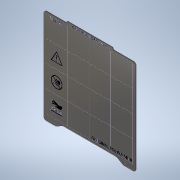
# Autodesk Inventor part: MINI-steel-sheet
Saved by Autodesk Inventor 2021 (Build 250183000, 183)
## iProperties
Created: 2019-07-15
Material: Všeobecné
Document SubType Name: Modeling
Density: 1 g/cm^3
Appearance: Ocel – leštěná
Project: ORIGINAL PRUSA MINI
Authority: Ing. Robert Turinský
Company: Prusa Development a.s.
Author: Ing. Robert Turinský
Title: MINI-steel-sheet
Revision Number: R4
Autodesk Inventor part; units mm, degrees
ref_plane "YZ Plane" through (0, 0, 0) normal (1, 0, 0) x (0, 1, 0)
ref_plane "XZ Plane" through (0, 0, 0) normal (0, 1, 0) x (-1, 0, 0)
ref_plane "XY Plane" through (0, 0, 0) normal (0, 0, 1) x (1, 0, 0)
sketch "Náčrt1" plane through (0, 0, 0) normal (0, 0, 1) x (1, 0, 0)
  line L0 (53.75, -94.15) -> (-53.75, -94.15)
  line L1 (-95, -97.15) -> (-95, 89.15)
  line L2 (95, 89.15) -> (95, -97.15)
  line L3 (0, -144.5745) -> (0, 138.3969) projected
  line L4 (-134.4497, 0) -> (134.4497, 0) projected
  arc A0 (95, 89.15) -> (90, 94.15) centre (90, 89.15) ccw
  arc A1 (-90, 94.15) -> (-95, 89.15) centre (-90, 89.15) ccw
  line L5 (-48.6171, 94.6805) -> (-47.2139, 97.3195)
  line L6 (-46.331, 97.85) -> (46.331, 97.85)
  line L7 (47.2139, 97.3195) -> (48.6171, 94.6805)
  line L8 (-90, 94.15) -> (-49.5, 94.15)
  line L9 (49.5, 94.15) -> (90, 94.15)
  line L10 (-90, -102.15) -> (-72.75, -102.15)
  line L11 (58.8398, -95.5422) -> (67.6602, -100.7578)
  line L12 (72.75, -102.15) -> (90, -102.15)
  arc A2 (-95, -97.15) -> (-90, -102.15) centre (-90, -97.15) ccw
  arc A3 (90, -102.15) -> (95, -97.15) centre (90, -97.15) ccw
  line L13 (-67.6602, -100.7578) -> (-58.8398, -95.5422)
  arc A4 (-72.75, -102.15) -> (-67.6602, -100.7578) centre (-72.75, -92.15) ccw
  arc A5 (-53.75, -94.15) -> (-58.8398, -95.5422) centre (-53.75, -104.15) ccw
  arc A6 (58.8398, -95.5422) -> (53.75, -94.15) centre (53.75, -104.15) ccw
  arc A7 (67.6602, -100.7578) -> (72.75, -102.15) centre (72.75, -92.15) ccw
  circle A8 centre (-72.75, -97.15) radius 1.75
  circle A9 centre (72.75, -97.15) radius 1.75
  arc A10 (-46.331, 97.85) -> (-47.2139, 97.3195) centre (-46.331, 96.85) ccw
  arc A11 (-49.5, 94.15) -> (-48.6171, 94.6805) centre (-49.5, 95.15) ccw
  arc A12 (48.6171, 94.6805) -> (49.5, 94.15) centre (49.5, 95.15) ccw
  arc A13 (47.2139, 97.3195) -> (46.331, 97.85) centre (46.331, 96.85) ccw
  arc A14 (48.6171, 94.6805) -> (49.5, 94.15) centre (49.5, 95.15) ccw
  point P0 (0, 0)
  point P1 (56.4853, -94.15)
  point P2 (-56.4853, -94.15)
  point P3 (-46.9318, 97.85)
  point P4 (46.9318, 97.85)
  point P5 (48.8991, 94.15)
  point P6 (-48.8991, 94.15)
  point P7 (-70.0147, -102.15)
  point P8 (70.0147, -102.15)
  dimension "d3" = 5
  dimension "d9" = 3.7
  dimension "d13" = 8
  dimension "d14" = 190
  dimension "d15" = 5
  dimension "d18" = 10
  dimension "d19" = 196.3
  dimension "d23" = 19
  dimension "d24" = 22.25
  dimension "d25" = 3.5
  dimension "d26" = 5
  dimension "d33" = 1
  dimension "d34" = 1
  dimension "d35" = 45.5
  dimension "d36" = 45.5
  dimension "d37" = 62
  dimension "d38" = 62
  constraints: 28 tangent, 26 point on circle, 24 end point, 19 point on line, 15 centre point, 9 equal radius, 3 horizontal, 3 parallel, 2 equal length, 2 vertical alignment, 1 collinear, 1 horizontal alignment, 1 perpendicular, 2 other
  measures "d3" radius of A0
  measures "d9" distance between parallel lines of L6 L9
  measures "d13" distance between parallel lines of L0 L10
  measures "d14" distance between parallel lines of L2 L1
  measures "d15" radius of A2
  measures "d18" radius of A4
  measures "d19" distance between parallel lines of L8 L10
  measures "d23" horizontal distance of A5.centre A4.centre
  measures "d24" distance from line of L1 A4.centre
  measures "d25" diameter of A8
  measures "d26" distance from line of L10 A8.centre
  measures "d33" radius of A10
  measures "d34" radius of A13
  measures "d35" distance from line of A11.centre L1
  measures "d36" distance from line of L2 A12.centre
  measures "d37" angle of L8 L5
  measures "d38" angle of L9 L7
extrude "Vysunutí1" add sketch "Náčrt1" along normal blind 1.4
sketch "Náčrt2" plane through (0, 0, 1.4) normal (0, 0, 1) x (1, 0, 0)
  line L0 (-90.5, 89.5) -> (89.5, 89.5)
  line L1 (89.5, 89.5) -> (89.5, -90.5)
  line L2 (89.5, -90.5) -> (-90.5, -90.5)
  line L3 (-90.5, -90.5) -> (-90.5, 89.5)
  line L4 (-90.4999, 89.4999) -> (89.4999, 89.4999)
  line L5 (89.4999, 89.4999) -> (89.4999, -90.4999)
  line L6 (89.4999, -90.4999) -> (-90.4999, -90.4999)
  line L7 (-90.4999, -90.4999) -> (-90.4999, 89.4999)
  point P0 (0, 0)
  dimension "d27" = 180
  dimension "d28" = 89.5
  dimension "d29" = 90.5
  dimension "d30" = 0.0001
  constraints: 16 end point, 4 parallel, 3 perpendicular, 1 horizontal, 3 other
  measures "d27" distance of L1.end L2.end
  measures "d28" distance from line of L1 point (0, 0)
  measures "d29" distance from line of L2 point (0, 0)
  measures "d30" distance between parallel lines of L3 L7
extrude "Vysunutí2" [suppressed]
sketch "Náčrt3" plane through (0, 0, 1.4) normal (0, 0, 1) x (1, 0, 0)
  line L0 (-95.75, 99.25) -> (95.75, 99.25) construction
  line L1 (95.75, 99.25) -> (95.75, -102.43) construction
  line L2 (95.75, -102.43) -> (-95.75, -102.43) construction
  line L3 (-95.75, -102.43) -> (-95.75, 99.25) construction
  point P0 (0, 0)
  point P1 (0, 177.5651)
  point P2 (0, 99.25)
  dimension "d63" = 191.5
  dimension "d84" = 99.25
  constraints: 2 vertical alignment, 1 midpoint, 2 other
  measures "d63" distance of L0.start L0.end
  measures "d84" distance from line of point (0, 0) L0
decal "Obtisk1"
equation "\"d3\" = d15"
equation "\"d34\" = d33"
equation "\"d36\" = d35"
equation "\"d38\" = d37"
